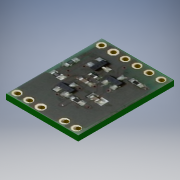
# Autodesk Inventor part: chip_gross
Saved by Autodesk Inventor 2017 (Build 210142000, 142)
## iProperties
Part Number: chip_gross
Material: Generisch
Document SubType Name: Modeling
Designer: Philomena-Theresa
Density: 1 g/cm^3
Appearance: Vorgabe
Author: Philomena-Theresa
Autodesk Inventor part; units mm, degrees
ref_plane "YZ Plane" through (0, 0, 0) normal (1, 0, 0) x (0, 1, 0)
ref_plane "XZ Plane" through (0, 0, 0) normal (0, 1, 0) x (-1, 0, 0)
ref_plane "XY Plane" through (0, 0, 0) normal (0, 0, 1) x (1, 0, 0)
sketch "Skizze1" plane through (0, 0, 0) normal (0, 0, 1) x (1, 0, 0)
  line L0 (-8.8926, 8.6829) -> (6.3574, 8.6829)
  line L1 (6.3574, 8.6829) -> (6.3574, -11.5571)
  line L2 (6.3574, -11.5571) -> (-8.8926, -11.5571)
  line L3 (-8.8926, -11.5571) -> (-8.8926, 8.6829)
  point P0 (0, 0)
  dimension "d0" = 15.25
  dimension "d1" = 20.24
  constraints: 8 end point, 2 parallel, 1 horizontal, 1 perpendicular
  measures "d0" distance of L1.end L2.end
  measures "d1" distance of L0.end L1.end
extrude "Extrusion2" add sketch "Skizze1" along normal blind 1.11
sketch "Skizze2" plane through (0, 0, 1.11) normal (0, 0, 1) x (1, 0, 0)
  line L0 (6.3574, 8.6829) -> (-8.8926, 8.6829) construction
  line L1 (-8.8926, 8.6829) -> (-8.8926, 7.3829) construction
  line L2 (-8.8926, 8.6829) -> (-8.8926, -11.5571) construction
  line L3 (-8.8926, 7.3829) -> (6.3574, 7.3829) construction
  line L4 (6.3574, -11.5571) -> (6.3574, 8.6829) construction
  line L5 (-8.8926, 7.3829) -> (-8.0926, 7.3829) construction
  line L6 (6.3574, 7.3829) -> (5.5574, 7.3829) construction
  line L7 (-8.0926, 7.3829) -> (-7.6426, 7.3829) construction
  circle A0 centre (-7.6426, 7.3829) radius 0.45
  circle A1 centre (-5.0926, 7.3829) radius 0.45
  circle A2 centre (-2.5426, 7.3829) radius 0.45
  circle A3 centre (0.0074, 7.3829) radius 0.45
  circle A4 centre (2.5574, 7.3829) radius 0.45
  circle A5 centre (5.1074, 7.3829) radius 0.45
  line L8 (-8.8926, -11.5571) -> (-8.8926, -10.2571) construction
  line L9 (-8.8926, -10.2571) -> (6.3574, -10.2571) construction
  line L10 (-8.8926, -10.2571) -> (-7.6426, -10.2571) construction
  circle A6 centre (-7.6426, -10.2571) radius 0.45
  circle A7 centre (-5.0926, -10.2571) radius 0.45
  line L11 (-6.3426, -10.2571) -> (8.9074, -10.2571) construction
  circle A8 centre (-2.5426, -10.2571) radius 0.45
  line L12 (-3.7926, -10.2571) -> (11.4574, -10.2571) construction
  circle A9 centre (0.0074, -10.2571) radius 0.45
  line L13 (-1.2426, -10.2571) -> (14.0074, -10.2571) construction
  circle A10 centre (2.5574, -10.2571) radius 0.45
  line L14 (1.3074, -10.2571) -> (16.5574, -10.2571) construction
  circle A11 centre (5.1074, -10.2571) radius 0.45
  line L15 (3.8574, -10.2571) -> (19.1074, -10.2571) construction
  line L16 (5.5574, 7.3829) -> (5.1074, 7.3829)
  point P0 (0, 0)
  dimension "d6" = 1.3
  dimension "d7" = 0.8
  dimension "d8" = 0.8
  dimension "d9" = 0.45
  dimension "d10" = 0.9
  dimension "d13" = 2.55
  dimension "d20" = 1.3
  dimension "d21" = 1.25
  dimension "d22" = 0.9
  dimension "d25" = 2.55
  dimension "d30" = 0.45
  constraints: 28 end point, 14 point on line, 12 centre point, 9 coincident, 2 horizontal, 2 perpendicular, 1 collinear, 39 other
  measures "d6" distance of L0.end L1.end
  measures "d7" distance of L1.end L5.end
  measures "d8" distance of L3.end L6.end
  measures "d9" distance of L7.start L7.end
  measures "d10" diameter of A0
  measures "d13" distance of A0.centre A1.centre
  measures "d20" distance of L2.end L8.end
  measures "d21" distance of L8.end L10.end
  measures "d22" diameter of A6
  measures "d25" distance of A6.centre A7.centre
  measures "d30" distance of L16.start L16.end
extrude "Extrusion3" cut sketch "Skizze2" against normal blind 1.11 contours A0 | A1 | A2 | A3 | A4 | A5 | A6 | A7 | A8 | A10 | A11
sketch "Skizze3" plane through (0, 0, 1.11) normal (0, 0, 1) x (1, 0, 0)
  line L0 (6.3574, 8.6829) -> (-8.8926, 8.6829) projected
  line L1 (-8.8926, 8.6829) -> (6.4364, 8.6229) construction
  line L2 (6.4364, 8.6229) -> (6.3574, -11.5571) construction
  line L3 (6.3574, -11.5571) -> (-8.9716, -11.4971) construction
  line L4 (-8.9716, -11.4971) -> (-8.8926, 8.6829) construction
  point P0 (0, 0)
  point P1 (-1.2676, 8.6829)
  point P2 (6.3574, -11.5571)
  constraints: 2 coincident, 1 midpoint, 2 other
decal "Aufkleber1"
sketch "Skizze4" plane through (0, 0, 0) normal (0, 0, -1) x (-1, 0, 0)
  line L0 (8.9962, -11.5571) -> (-6.461, -11.5571) construction
  line L1 (-6.461, -11.5571) -> (-6.461, 8.6829) construction
  line L2 (-6.461, 8.6829) -> (8.9962, 8.6829) construction
  line L3 (8.9962, 8.6829) -> (8.9962, -11.5571) construction
  line L4 (-6.3574, -11.5571) -> (8.8926, -11.5571) projected
  line L5 (8.8926, 8.6829) -> (-6.3574, 8.6829) projected
  point P0 (0, 0)
  point P1 (1.2676, -11.5571)
  point P2 (1.2676, 8.6829)
  constraints: 4 midpoint, 2 other
decal "Aufkleber2"
